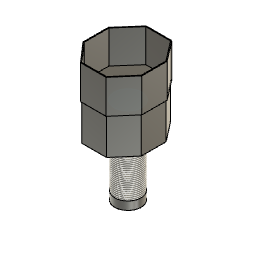
idea1 v1 (Autodesk Fusion 360 design; units mm, degrees)
Autodesk Fusion 360 part; units mm, degrees
sketch "Schizzo1" plane through (0, 0, 0) normal (0, 0, 1) x (1, 0, 0)
  line L0 (-15, 20) -> (15, 20)
  line L1 (15, 20) -> (33.3235, -3.754)
  line L2 (33.3235, -3.754) -> (33.3235, -33.754)
  line L3 (33.3235, -33.754) -> (13.7304, -56.4721)
  line L4 (13.7304, -56.4721) -> (-16.2696, -56.4721)
  line L5 (-16.2696, -56.4721) -> (-35.9903, -33.8647)
  line L6 (-35.9903, -33.8647) -> (-35.9903, -3.8647)
  line L7 (-35.9903, -3.8647) -> (-15, 20)
  dimension "d1" = 30
  dimension "d2" = 30
  dimension "d3" = 30
  dimension "d4" = 30
  dimension "d5" = 30
  dimension "d6" = 30
  constraint horizontal L0
  constraint perpendicular L0 L2
  constraint horizontal L4
  constraint vertical L6
  measures "d1" distance of L0.end L1.end
  measures "d2" distance of L1.end L2.end
  measures "d3" distance of L2.end L3.end
  measures "d4" distance of L3.end L4.end
  measures "d5" distance of L4.end L5.end
  measures "d6" distance of L5.end L6.end
extrude "Estrusione1" add sketch "Schizzo1" along normal blind 75 makes body 1
ref_plane "Piano di lavoro1" through (-1.3334, -18.236, 35) normal (0, 0, -1) x (-1, 0, 0)
split "Dividi1" by plane through (-1.3334, -18.236, 35) normal (0, 0, -1) bodies 1 makes body 2 at (-12.8857, -23.8278, 0)
shell "Svuotamento1" thickness 1 outward yes removed faces 1 at (-12.8857, -23.8278, 75) on bodies 1
hole "Foratura1" at (1.1863, -17.8776, 0) direction (0, 0, 1) diameter 33.526 depth 25 tip angle 180 bodies 2
thread "Filettatura1" "ISO Metric profile 35.0 M35x1.5 6H"
sketch "Schizzo2" plane through (0, 0, 25) normal (0, 0, -1) x (1, 0, 0)
  circle A0 centre (1.1863, 17.8776) radius 16.763
sketch "Schizzo3" plane through (0, 0, 0) normal (0, 0, -1) x (1, 0, 0)
  circle A0 centre (1.1863, 17.8776) radius 16.763
  line L0 (-35.9903, 33.8647) -> (-35.9903, 3.8647)
  line L1 (-35.9903, 3.8647) -> (-15, -20)
  line L2 (-15, -20) -> (15, -20)
  line L3 (15, -20) -> (33.3235, 3.754)
  line L4 (33.3235, 3.754) -> (33.3235, 33.754)
  line L5 (33.3235, 33.754) -> (13.7304, 56.4721)
  line L6 (13.7304, 56.4721) -> (-16.2696, 56.4721)
  line L7 (-16.2696, 56.4721) -> (-35.9903, 33.8647)
  circle A1 centre (1.1863, 17.8776) radius 16.763
  constraint concentric A0 A1
extrude "Estrusione2" add sketch "Schizzo3" along normal blind 70 separate body contours A0 A1 makes body 3
thread "Filettatura2" "ISO Metric profile 32.0 M32x2 6g" major diameter 31.822 minor diameter 29.5289 pitch 2 angle 60 resizes the face on face at (17.866, -16.2086, -46.6667) on bodies 3
sketch "Schizzo4" plane through (0, 0, -70) normal (0, 0, -1) x (1, 0, 0)
  circle A0 centre (1.1863, 17.8776) radius 15.911
  line L0 (-5, 30) -> (5, 30)
  line L1 (5, 30) -> (5, 5)
  line L2 (5, 5) -> (-5, 5)
  line L3 (-5, 5) -> (-5, 30)
  constraint horizontal L0
  constraint vertical L1
  constraint horizontal L2
  constraint vertical L3
sketch "Schizzo5" plane through (0, 0, -70) normal (0, 0, -1) x (1, 0, 0)
  circle A0 centre (1.1863, 17.8776) radius 15.911
extrude "Estrusione3" cut sketch "Schizzo4" against normal blind 75 contours L0 L1 L2 L3 bodies 3
extrude "Estrusione4" add 1 faces at (-1.2837, -49.1325, 0) along direction (0, 0, -1) blind 10 on bodies 2 bodies 2
sketch "Schizzo6" plane through (0, 0, 0) normal (0, 0, 1) x (1, 0, 0)
extrude "Estrusione5" add sketch "Schizzo5" along normal blind 10 separate body makes body 4
hole "Foratura2" at (5.9036, -13.9599, -80) direction (0, 0, 1) diameter 10 depth 5 tip angle 118 bodies 4
hole "Foratura3" at (-2.7621, -19.8067, -80) direction (0, 0, 1) diameter 10 depth 5 tip angle 118 bodies 4
named bodies: "Corpo racchetta", "Corpo sotto racchetta", "Corpo per PCB", "Tappo con pulsante LED e pulsante ON/OFF"
